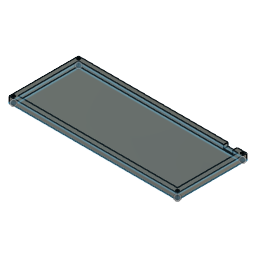
Keyboard Assembled (Autodesk Fusion 360 archive; units mm, degrees)
design "KeyboardBottom"
part number: 2026-01-12-19-14-13-415
Autodesk Fusion 360 part; units mm, degrees
(part 1 of 2)
sketch "Sketch1" plane through (0, 0, 0) normal (0, 0, 1) x (1, 0, 0)
  line L0 (0, 250) -> (351, 250)
  line L1 (351, 250) -> (351, 383)
  line L2 (351, 383) -> (0, 383)
  line L3 (0, 383) -> (0, 250)
  line L4 (-9.5, 392.5) -> (361.5, 392.5)
  line L5 (361.5, 392.5) -> (361.5, 239.5)
  line L6 (361.5, 239.5) -> (-9.5, 239.5)
  line L7 (-9.5, 239.5) -> (-9.5, 392.5)
  circle A0 centre (-4.5, 244.5) radius 1.7
  circle A1 centre (356.5, 244.5) radius 1.7
  circle A2 centre (-4.5, 387.5) radius 1.7
  circle A3 centre (356.5, 387.5) radius 1.7
  circle A4 centre (-4.5, 387.5) radius 3
  circle A5 centre (356.5, 244.5) radius 3
  circle A6 centre (-4.5, 244.5) radius 3
  circle A7 centre (356.5, 387.5) radius 3
  dimension "d1" = 351
  dimension "d2" = 133
  dimension "d3" = 371
  dimension "d4" = 153
  dimension "d5" = 9.5
  dimension "d10" = 9.5
  dimension "d11" = 3.4
  dimension "d12" = 5
  dimension "d13" = 5
  dimension "d14" = 3.4
  dimension "d15" = 5
  dimension "d16" = 5
  dimension "d17" = 3.4
  dimension "d18" = 5
  dimension "d19" = 5
  dimension "d21" = 5
  dimension "d22" = 5
  dimension "d23" = 6
  dimension "d24" = 6
  dimension "d25" = 6
  dimension "d26" = 6
  constraint horizontal L0
  constraint vertical L1
  constraint horizontal L2
  constraint vertical L3
  constraint horizontal L4
  constraint vertical L5
  constraint horizontal L6
  constraint vertical L7
  constraint coincident A2.centre A4.centre
  constraint coincident A0.centre A6.centre
  constraint coincident A1.centre A5.centre
  constraint coincident A3.centre A7.centre
  measures "d1" distance of L0.start L0.end
  measures "d2" distance of L0.start L2.end
  measures "d3" distance of L4.start L4.end
  measures "d4" distance of L4.start L6.end
  measures "d5" distance of L3 L7
  measures "d10" distance of L2 L4
  measures "d11" diameter of A0
  measures "d12" distance of L6 A0.centre
  measures "d13" distance of L7 A0.centre
  measures "d14" diameter of A1
  measures "d15" distance of L6 A1.centre
  measures "d16" distance of L5 A1.centre
  measures "d17" diameter of A2
  measures "d18" distance of L4 A2.centre
  measures "d19" distance of L7 A2.centre
  measures "d21" distance of L4 A3.centre
  measures "d22" distance of L5 A3.centre
  measures "d23" diameter of A4
  measures "d24" diameter of A5
  measures "d25" diameter of A6
  measures "d26" diameter of A7
extrude "Extrude1" add sketch "Sketch1" along normal blind 10 from surface at 3.1 contours A4 | A5 | A6 | A7 makes body 1 at (-1.5928, 245.2403, 9.7667) makes body 2 at (357.3125, 247.3879, 9.7667) makes body 3 at (-7.0599, 389.0643, 9.7667) makes body 4 at (355.1314, 384.8304, 6.4333)
extrude "Extrude2" add sketch "Sketch1" along normal blind 13 contours L4 L5 L6 L7 bodies 1 2 3 4
extrude "Extrude3" add sketch "Sketch1" along normal blind 3 contours L0 L1 L2 L3 bodies 1
sketch "Sketch2" plane through (0, 0, 13) normal (0, 0, 1) x (-1, 0, 0)
  line L0 (0, -250) -> (0, -383)
  line L1 (0, -383) -> (-351, -383)
  line L2 (-351, -383) -> (-351, -250)
  line L3 (-351, -250) -> (0, -250)
  circle A0 centre (-356.5, -244.5) radius 3
  circle A1 centre (4.5, -244.5) radius 3
  circle A2 centre (4.5, -387.5) radius 3
  circle A3 centre (-356.5, -387.5) radius 3
  line L4 (9.5, -239.5) -> (-361.5, -239.5)
  line L5 (-361.5, -239.5) -> (-361.5, -392.5)
  line L6 (-361.5, -392.5) -> (9.5, -392.5)
  line L7 (9.5, -392.5) -> (9.5, -239.5)
sketch "Sketch3" plane through (0, 0, 13) normal (0, 0, 1) x (-1, 0, 0)
  line L0 (2440, -1230) -> (2470, -1230)
  line L1 (2470, -1230) -> (2470, -1260)
  line L2 (2470, -1260) -> (2440, -1260)
  line L3 (2440, -1260) -> (2440, -1230)
  constraint horizontal L0
  constraint vertical L1
  constraint horizontal L2
  constraint vertical L3
sketch "Sketch4" plane through (0, 0, 0) normal (1, 0, 0) x (0, 1, 0)
sketch "Sketch5" plane through (0, 0, 0) normal (0, 0, 1) x (1, 0, 0)
extrude "Extrude4" cut sketch "Sketch3" against normal blind 7.5 bodies 1
sketch "Sketch6" plane through (0, 0, 13) normal (0, 0, 1) x (-1, 0, 0)
  line L0 (-320, -400) -> (-340, -400)
  line L1 (-340, -400) -> (-340, -380)
  line L2 (-340, -380) -> (-320, -380)
  line L3 (-320, -380) -> (-320, -400)
  constraint horizontal L0
  constraint vertical L1
  constraint horizontal L2
  constraint vertical L3
extrude "Extrude5" cut sketch "Sketch6" against normal blind 7.5 bodies 1

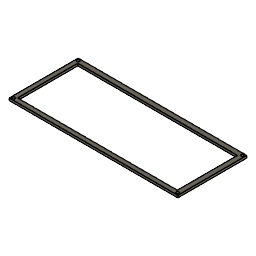
design "KeyboardBezel"
part number: 2026-01-27-16-23-20-670
Autodesk Fusion 360 part; units mm, degrees
sketch "Sketch1" plane through (0, 0, 0) normal (0, 0, 1) x (1, 0, 0)
  line L0 (0, 0) -> (-371, 0)
  line L1 (-371, 0) -> (-371, 152)
  line L2 (-371, 152) -> (0, 152)
  line L3 (0, 152) -> (0, 0)
  circle A0 centre (-366, 147) radius 1.7
  circle A1 centre (-5, 5) radius 1.7
  circle A2 centre (-366, 5) radius 1.7
  circle A3 centre (-5, 147) radius 1.7
  circle A4 centre (-366, 147) radius 3
  circle A5 centre (-5, 5) radius 3
  circle A6 centre (-366, 5) radius 3
  circle A7 centre (-5, 147) radius 3
  dimension "d1" = 371
  dimension "d2" = 152
  dimension "d3" = 3.4
  dimension "d4" = 5
  dimension "d5" = 5
  dimension "d6" = 3.4
  dimension "d7" = 3.4
  dimension "d8" = 3.4
  dimension "d9" = 5
  dimension "d10" = 5
  dimension "d11" = 5
  dimension "d12" = 5
  dimension "d13" = 5
  dimension "d14" = 5
  dimension "d15" = 6
  dimension "d16" = 6
  dimension "d17" = 6
  dimension "d18" = 6
  constraint horizontal L0
  constraint vertical L1
  constraint horizontal L2
  constraint vertical L3
  constraint coincident L0.start L3.end
  constraint coincident A1.centre A5.centre
  constraint coincident A3.centre A7.centre
  constraint coincident A0.centre A4.centre
  constraint coincident A2.centre A6.centre
  measures "d1" distance of L0.start L0.end
  measures "d2" distance of L0.start L2.end
  measures "d3" diameter of A0
  measures "d4" distance of L2 A0.centre
  measures "d5" distance of L1 A0.centre
  measures "d6" diameter of A1
  measures "d7" diameter of A2
  measures "d8" diameter of A3
  measures "d9" distance of L0 A2.centre
  measures "d10" distance of L1 A2.centre
  measures "d11" distance of L0 A1.centre
  measures "d12" distance of L3 A1.centre
  measures "d13" distance of L2 A3.centre
  measures "d14" distance of L3 A3.centre
  measures "d15" diameter of A4
  measures "d16" diameter of A5
  measures "d17" diameter of A6
  measures "d18" diameter of A7
sketch "Sketch2" plane through (0, 0, 0) normal (0, 0, 1) x (1, 0, 0)
  line L0 (-361.5, 141.5) -> (-10.5, 141.5)
  line L1 (-10.5, 141.5) -> (-10.5, 9.5)
  line L2 (-10.5, 9.5) -> (-361.5, 9.5)
  line L3 (-361.5, 9.5) -> (-361.5, 141.5)
  line L4 (0, 0) -> (-371, 0)
  line L5 (-371, 0) -> (-371, 152)
  dimension "d19" = 351
  dimension "d20" = 132
  dimension "d21" = 9.5
  dimension "d22" = 9.5
  constraint horizontal L0
  constraint vertical L1
  constraint horizontal L2
  constraint vertical L3
  measures "d19" distance of L0.start L0.end
  measures "d20" distance of L0.start L2.end
  measures "d21" distance of L2 L4
  measures "d22" distance of L3 L5
extrude "Extrude1" add sketch "Sketch1" along normal blind 5 contours L0 L1 L2 L3
extrude "Extrude2" cut sketch "Sketch2" along normal blind 10

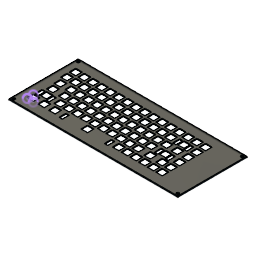
design "KeyboardPlate"
part number: 2026-01-21-16-41-26-618
Autodesk Fusion 360 part; units mm, degrees
sketch "plate-2026-01-22T00_34_46.063Z" plane through (0, 0, 0) normal (0, 0, 1) x (1, 0, 0)
  line L0 (3.025, -2.525) -> (16.025, -2.525)
  line L1 (3.025, -16.525) -> (16.025, -16.525)
  line L2 (2.525, -3.025) -> (2.525, -16.025)
  line L3 (16.525, -3.025) -> (16.525, -16.025)
  arc A0 (3.025, -2.525) -> (2.525, -3.025) centre (3.025, -3.025) ccw
  arc A1 (16.525, -3.025) -> (16.025, -2.525) centre (16.025, -3.025) ccw
  arc A2 (2.525, -16.025) -> (3.025, -16.525) centre (3.025, -16.025) ccw
  arc A3 (16.025, -16.525) -> (16.525, -16.025) centre (16.025, -16.025) ccw
  line L4 (22.075, -2.525) -> (35.075, -2.525)
  line L5 (22.075, -16.525) -> (35.075, -16.525)
  line L6 (21.575, -3.025) -> (21.575, -16.025)
  line L7 (35.575, -3.025) -> (35.575, -16.025)
  arc A4 (22.075, -2.525) -> (21.575, -3.025) centre (22.075, -3.025) ccw
  arc A5 (35.575, -3.025) -> (35.075, -2.525) centre (35.075, -3.025) ccw
  arc A6 (21.575, -16.025) -> (22.075, -16.525) centre (22.075, -16.025) ccw
  arc A7 (35.075, -16.525) -> (35.575, -16.025) centre (35.075, -16.025) ccw
  line L8 (41.125, -2.525) -> (54.125, -2.525)
  line L9 (41.125, -16.525) -> (54.125, -16.525)
  line L10 (40.625, -3.025) -> (40.625, -16.025)
  line L11 (54.625, -3.025) -> (54.625, -16.025)
  arc A8 (41.125, -2.525) -> (40.625, -3.025) centre (41.125, -3.025) ccw
  arc A9 (54.625, -3.025) -> (54.125, -2.525) centre (54.125, -3.025) ccw
  arc A10 (40.625, -16.025) -> (41.125, -16.525) centre (41.125, -16.025) ccw
  arc A11 (54.125, -16.525) -> (54.625, -16.025) centre (54.125, -16.025) ccw
  line L12 (60.175, -2.525) -> (73.175, -2.525)
  line L13 (60.175, -16.525) -> (73.175, -16.525)
  line L14 (59.675, -3.025) -> (59.675, -16.025)
  line L15 (73.675, -3.025) -> (73.675, -16.025)
  arc A12 (60.175, -2.525) -> (59.675, -3.025) centre (60.175, -3.025) ccw
  arc A13 (73.675, -3.025) -> (73.175, -2.525) centre (73.175, -3.025) ccw
  arc A14 (59.675, -16.025) -> (60.175, -16.525) centre (60.175, -16.025) ccw
  arc A15 (73.175, -16.525) -> (73.675, -16.025) centre (73.175, -16.025) ccw
  line L16 (79.225, -2.525) -> (92.225, -2.525)
  line L17 (79.225, -16.525) -> (92.225, -16.525)
  line L18 (78.725, -3.025) -> (78.725, -16.025)
  line L19 (92.725, -3.025) -> (92.725, -16.025)
  arc A16 (79.225, -2.525) -> (78.725, -3.025) centre (79.225, -3.025) ccw
  arc A17 (92.725, -3.025) -> (92.225, -2.525) centre (92.225, -3.025) ccw
  arc A18 (78.725, -16.025) -> (79.225, -16.525) centre (79.225, -16.025) ccw
  arc A19 (92.225, -16.525) -> (92.725, -16.025) centre (92.225, -16.025) ccw
  line L20 (98.275, -2.525) -> (111.275, -2.525)
  line L21 (98.275, -16.525) -> (111.275, -16.525)
  line L22 (97.775, -3.025) -> (97.775, -16.025)
  line L23 (111.775, -3.025) -> (111.775, -16.025)
  arc A20 (98.275, -2.525) -> (97.775, -3.025) centre (98.275, -3.025) ccw
  arc A21 (111.775, -3.025) -> (111.275, -2.525) centre (111.275, -3.025) ccw
  arc A22 (97.775, -16.025) -> (98.275, -16.525) centre (98.275, -16.025) ccw
  arc A23 (111.275, -16.525) -> (111.775, -16.025) centre (111.275, -16.025) ccw
  line L24 (117.325, -2.525) -> (130.325, -2.525)
  line L25 (117.325, -16.525) -> (130.325, -16.525)
  line L26 (116.825, -3.025) -> (116.825, -16.025)
  line L27 (130.825, -3.025) -> (130.825, -16.025)
  arc A24 (117.325, -2.525) -> (116.825, -3.025) centre (117.325, -3.025) ccw
  arc A25 (130.825, -3.025) -> (130.325, -2.525) centre (130.325, -3.025) ccw
  arc A26 (116.825, -16.025) -> (117.325, -16.525) centre (117.325, -16.025) ccw
  arc A27 (130.325, -16.525) -> (130.825, -16.025) centre (130.325, -16.025) ccw
  line L28 (136.375, -2.525) -> (149.375, -2.525)
  line L29 (136.375, -16.525) -> (149.375, -16.525)
  line L30 (135.875, -3.025) -> (135.875, -16.025)
  line L31 (149.875, -3.025) -> (149.875, -16.025)
  arc A28 (136.375, -2.525) -> (135.875, -3.025) centre (136.375, -3.025) ccw
  arc A29 (149.875, -3.025) -> (149.375, -2.525) centre (149.375, -3.025) ccw
  arc A30 (135.875, -16.025) -> (136.375, -16.525) centre (136.375, -16.025) ccw
  arc A31 (149.375, -16.525) -> (149.875, -16.025) centre (149.375, -16.025) ccw
  line L32 (155.425, -2.525) -> (168.425, -2.525)
  line L33 (155.425, -16.525) -> (168.425, -16.525)
  line L34 (154.925, -3.025) -> (154.925, -16.025)
  line L35 (168.925, -3.025) -> (168.925, -16.025)
  arc A32 (155.425, -2.525) -> (154.925, -3.025) centre (155.425, -3.025) ccw
  arc A33 (168.925, -3.025) -> (168.425, -2.525) centre (168.425, -3.025) ccw
  arc A34 (154.925, -16.025) -> (155.425, -16.525) centre (155.425, -16.025) ccw
  arc A35 (168.425, -16.525) -> (168.925, -16.025) centre (168.425, -16.025) ccw
  line L36 (174.475, -2.525) -> (187.475, -2.525)
  line L37 (174.475, -16.525) -> (187.475, -16.525)
  line L38 (173.975, -3.025) -> (173.975, -16.025)
  line L39 (187.975, -3.025) -> (187.975, -16.025)
  arc A36 (174.475, -2.525) -> (173.975, -3.025) centre (174.475, -3.025) ccw
  arc A37 (187.975, -3.025) -> (187.475, -2.525) centre (187.475, -3.025) ccw
  arc A38 (173.975, -16.025) -> (174.475, -16.525) centre (174.475, -16.025) ccw
  arc A39 (187.475, -16.525) -> (187.975, -16.025) centre (187.475, -16.025) ccw
  line L40 (193.525, -2.525) -> (206.525, -2.525)
  line L41 (193.525, -16.525) -> (206.525, -16.525)
  line L42 (193.025, -3.025) -> (193.025, -16.025)
  line L43 (207.025, -3.025) -> (207.025, -16.025)
  arc A40 (193.525, -2.525) -> (193.025, -3.025) centre (193.525, -3.025) ccw
  arc A41 (207.025, -3.025) -> (206.525, -2.525) centre (206.525, -3.025) ccw
  arc A42 (193.025, -16.025) -> (193.525, -16.525) centre (193.525, -16.025) ccw
  arc A43 (206.525, -16.525) -> (207.025, -16.025) centre (206.525, -16.025) ccw
  line L44 (212.575, -2.525) -> (225.575, -2.525)
  line L45 (212.575, -16.525) -> (225.575, -16.525)
  line L46 (212.075, -3.025) -> (212.075, -16.025)
  line L47 (226.075, -3.025) -> (226.075, -16.025)
  arc A44 (212.575, -2.525) -> (212.075, -3.025) centre (212.575, -3.025) ccw
  arc A45 (226.075, -3.025) -> (225.575, -2.525) centre (225.575, -3.025) ccw
  arc A46 (212.075, -16.025) -> (212.575, -16.525) centre (212.575, -16.025) ccw
  arc A47 (225.575, -16.525) -> (226.075, -16.025) centre (225.575, -16.025) ccw
  line L48 (231.625, -2.525) -> (244.625, -2.525)
  line L49 (231.625, -16.525) -> (244.625, -16.525)
  line L50 (231.125, -3.025) -> (231.125, -16.025)
  line L51 (245.125, -3.025) -> (245.125, -16.025)
  arc A48 (231.625, -2.525) -> (231.125, -3.025) centre (231.625, -3.025) ccw
  arc A49 (245.125, -3.025) -> (244.625, -2.525) centre (244.625, -3.025) ccw
  arc A50 (231.125, -16.025) -> (231.625, -16.525) centre (231.625, -16.025) ccw
  arc A51 (244.625, -16.525) -> (245.125, -16.025) centre (244.625, -16.025) ccw
  line L52 (250.675, -2.525) -> (263.675, -2.525)
  line L53 (250.675, -16.525) -> (263.675, -16.525)
  line L54 (250.175, -3.025) -> (250.175, -16.025)
  line L55 (264.175, -3.025) -> (264.175, -16.025)
  arc A52 (250.675, -2.525) -> (250.175, -3.025) centre (250.675, -3.025) ccw
  arc A53 (264.175, -3.025) -> (263.675, -2.525) centre (263.675, -3.025) ccw
  arc A54 (250.175, -16.025) -> (250.675, -16.525) centre (250.675, -16.025) ccw
  arc A55 (263.675, -16.525) -> (264.175, -16.025) centre (263.675, -16.025) ccw
  line L56 (269.725, -2.525) -> (282.725, -2.525)
  line L57 (269.725, -16.525) -> (282.725, -16.525)
  line L58 (269.225, -3.025) -> (269.225, -16.025)
  line L59 (283.225, -3.025) -> (283.225, -16.025)
  arc A56 (269.725, -2.525) -> (269.225, -3.025) centre (269.725, -3.025) ccw
  arc A57 (283.225, -3.025) -> (282.725, -2.525) centre (282.725, -3.025) ccw
  arc A58 (269.225, -16.025) -> (269.725, -16.525) centre (269.725, -16.025) ccw
  arc A59 (282.725, -16.525) -> (283.225, -16.025) centre (282.725, -16.025) ccw
  line L60 (288.775, -2.525) -> (301.775, -2.525)
  line L61 (288.775, -16.525) -> (301.775, -16.525)
  line L62 (288.275, -3.025) -> (288.275, -16.025)
  line L63 (302.275, -3.025) -> (302.275, -16.025)
  arc A60 (288.775, -2.525) -> (288.275, -3.025) centre (288.775, -3.025) ccw
  arc A61 (302.275, -3.025) -> (301.775, -2.525) centre (301.775, -3.025) ccw
  arc A62 (288.275, -16.025) -> (288.775, -16.525) centre (288.775, -16.025) ccw
  arc A63 (301.775, -16.525) -> (302.275, -16.025) centre (301.775, -16.025) ccw
  line L64 (3.025, -21.575) -> (16.025, -21.575)
  line L65 (3.025, -35.575) -> (16.025, -35.575)
  line L66 (2.525, -22.075) -> (2.525, -35.075)
  line L67 (16.525, -22.075) -> (16.525, -35.075)
  arc A64 (3.025, -21.575) -> (2.525, -22.075) centre (3.025, -22.075) ccw
  arc A65 (16.525, -22.075) -> (16.025, -21.575) centre (16.025, -22.075) ccw
  arc A66 (2.525, -35.075) -> (3.025, -35.575) centre (3.025, -35.075) ccw
  arc A67 (16.025, -35.575) -> (16.525, -35.075) centre (16.025, -35.075) ccw
  line L68 (22.075, -21.575) -> (35.075, -21.575)
  line L69 (22.075, -35.575) -> (35.075, -35.575)
  line L70 (21.575, -22.075) -> (21.575, -35.075)
  line L71 (35.575, -22.075) -> (35.575, -35.075)
  arc A68 (22.075, -21.575) -> (21.575, -22.075) centre (22.075, -22.075) ccw
  arc A69 (35.575, -22.075) -> (35.075, -21.575) centre (35.075, -22.075) ccw
  arc A70 (21.575, -35.075) -> (22.075, -35.575) centre (22.075, -35.075) ccw
  arc A71 (35.075, -35.575) -> (35.575, -35.075) centre (35.075, -35.075) ccw
  line L72 (41.125, -21.575) -> (54.125, -21.575)
  line L73 (41.125, -35.575) -> (54.125, -35.575)
  line L74 (40.625, -22.075) -> (40.625, -35.075)
  line L75 (54.625, -22.075) -> (54.625, -35.075)
  arc A72 (41.125, -21.575) -> (40.625, -22.075) centre (41.125, -22.075) ccw
  arc A73 (54.625, -22.075) -> (54.125, -21.575) centre (54.125, -22.075) ccw
  arc A74 (40.625, -35.075) -> (41.125, -35.575) centre (41.125, -35.075) ccw
  arc A75 (54.125, -35.575) -> (54.625, -35.075) centre (54.125, -35.075) ccw
  line L76 (60.175, -21.575) -> (73.175, -21.575)
  line L77 (60.175, -35.575) -> (73.175, -35.575)
  line L78 (59.675, -22.075) -> (59.675, -35.075)
  line L79 (73.675, -22.075) -> (73.675, -35.075)
  arc A76 (60.175, -21.575) -> (59.675, -22.075) centre (60.175, -22.075) ccw
  arc A77 (73.675, -22.075) -> (73.175, -21.575) centre (73.175, -22.075) ccw
  arc A78 (59.675, -35.075) -> (60.175, -35.575) centre (60.175, -35.075) ccw
  arc A79 (73.175, -35.575) -> (73.675, -35.075) centre (73.175, -35.075) ccw
  line L80 (79.225, -21.575) -> (92.225, -21.575)
  line L81 (79.225, -35.575) -> (92.225, -35.575)
  line L82 (78.725, -22.075) -> (78.725, -35.075)
  line L83 (92.725, -22.075) -> (92.725, -35.075)
  arc A80 (79.225, -21.575) -> (78.725, -22.075) centre (79.225, -22.075) ccw
  arc A81 (92.725, -22.075) -> (92.225, -21.575) centre (92.225, -22.075) ccw
  arc A82 (78.725, -35.075) -> (79.225, -35.575) centre (79.225, -35.075) ccw
  arc A83 (92.225, -35.575) -> (92.725, -35.075) centre (92.225, -35.075) ccw
  line L84 (98.275, -21.575) -> (111.275, -21.575)
  line L85 (98.275, -35.575) -> (111.275, -35.575)
  line L86 (97.775, -22.075) -> (97.775, -35.075)
  line L87 (111.775, -22.075) -> (111.775, -35.075)
  arc A84 (98.275, -21.575) -> (97.775, -22.075) centre (98.275, -22.075) ccw
  arc A85 (111.775, -22.075) -> (111.275, -21.575) centre (111.275, -22.075) ccw
  arc A86 (97.775, -35.075) -> (98.275, -35.575) centre (98.275, -35.075) ccw
  arc A87 (111.275, -35.575) -> (111.775, -35.075) centre (111.275, -35.075) ccw
  line L88 (117.325, -21.575) -> (130.325, -21.575)
  line L89 (117.325, -35.575) -> (130.325, -35.575)
  line L90 (116.825, -22.075) -> (116.825, -35.075)
  line L91 (130.825, -22.075) -> (130.825, -35.075)
  arc A88 (117.325, -21.575) -> (116.825, -22.075) centre (117.325, -22.075) ccw
  arc A89 (130.825, -22.075) -> (130.325, -21.575) centre (130.325, -22.075) ccw
  arc A90 (116.825, -35.075) -> (117.325, -35.575) centre (117.325, -35.075) ccw
  arc A91 (130.325, -35.575) -> (130.825, -35.075) centre (130.325, -35.075) ccw
  line L92 (136.375, -21.575) -> (149.375, -21.575)
  line L93 (136.375, -35.575) -> (149.375, -35.575)
  line L94 (135.875, -22.075) -> (135.875, -35.075)
  line L95 (149.875, -22.075) -> (149.875, -35.075)
  arc A92 (136.375, -21.575) -> (135.875, -22.075) centre (136.375, -22.075) ccw
  arc A93 (149.875, -22.075) -> (149.375, -21.575) centre (149.375, -22.075) ccw
  arc A94 (135.875, -35.075) -> (136.375, -35.575) centre (136.375, -35.075) ccw
  arc A95 (149.375, -35.575) -> (149.875, -35.075) centre (149.375, -35.075) ccw
  line L96 (155.425, -21.575) -> (168.425, -21.575)
  line L97 (155.425, -35.575) -> (168.425, -35.575)
  line L98 (154.925, -22.075) -> (154.925, -35.075)
  line L99 (168.925, -22.075) -> (168.925, -35.075)
  arc A96 (155.425, -21.575) -> (154.925, -22.075) centre (155.425, -22.075) ccw
  arc A97 (168.925, -22.075) -> (168.425, -21.575) centre (168.425, -22.075) ccw
  arc A98 (154.925, -35.075) -> (155.425, -35.575) centre (155.425, -35.075) ccw
  arc A99 (168.425, -35.575) -> (168.925, -35.075) centre (168.425, -35.075) ccw
  line L100 (174.475, -21.575) -> (187.475, -21.575)
  line L101 (174.475, -35.575) -> (187.475, -35.575)
  line L102 (173.975, -22.075) -> (173.975, -35.075)
  line L103 (187.975, -22.075) -> (187.975, -35.075)
  arc A100 (174.475, -21.575) -> (173.975, -22.075) centre (174.475, -22.075) ccw
  arc A101 (187.975, -22.075) -> (187.475, -21.575) centre (187.475, -22.075) ccw
  arc A102 (173.975, -35.075) -> (174.475, -35.575) centre (174.475, -35.075) ccw
  arc A103 (187.475, -35.575) -> (187.975, -35.075) centre (187.475, -35.075) ccw
  line L104 (193.525, -21.575) -> (206.525, -21.575)
  line L105 (193.525, -35.575) -> (206.525, -35.575)
  line L106 (193.025, -22.075) -> (193.025, -35.075)
  line L107 (207.025, -22.075) -> (207.025, -35.075)
  arc A104 (193.525, -21.575) -> (193.025, -22.075) centre (193.525, -22.075) ccw
  arc A105 (207.025, -22.075) -> (206.525, -21.575) centre (206.525, -22.075) ccw
  arc A106 (193.025, -35.075) -> (193.525, -35.575) centre (193.525, -35.075) ccw
  arc A107 (206.525, -35.575) -> (207.025, -35.075) centre (206.525, -35.075) ccw
  line L108 (212.575, -21.575) -> (225.575, -21.575)
  line L109 (212.575, -35.575) -> (225.575, -35.575)
  line L110 (212.075, -22.075) -> (212.075, -35.075)
  line L111 (226.075, -22.075) -> (226.075, -35.075)
  arc A108 (212.575, -21.575) -> (212.075, -22.075) centre (212.575, -22.075) ccw
  arc A109 (226.075, -22.075) -> (225.575, -21.575) centre (225.575, -22.075) ccw
  arc A110 (212.075, -35.075) -> (212.575, -35.575) centre (212.575, -35.075) ccw
  arc A111 (225.575, -35.575) -> (226.075, -35.075) centre (225.575, -35.075) ccw
  line L112 (231.625, -21.575) -> (244.625, -21.575)
  line L113 (231.625, -35.575) -> (244.625, -35.575)
  line L114 (231.125, -22.075) -> (231.125, -35.075)
  line L115 (245.125, -22.075) -> (245.125, -35.075)
  arc A112 (231.625, -21.575) -> (231.125, -22.075) centre (231.625, -22.075) ccw
  arc A113 (245.125, -22.075) -> (244.625, -21.575) centre (244.625, -22.075) ccw
  arc A114 (231.125, -35.075) -> (231.625, -35.575) centre (231.625, -35.075) ccw
  arc A115 (244.625, -35.575) -> (245.125, -35.075) centre (244.625, -35.075) ccw
  line L116 (260.2, -21.575) -> (273.2, -21.575)
  line L117 (260.2, -35.575) -> (273.2, -35.575)
  line L118 (259.7, -22.075) -> (259.7, -35.075)
  line L119 (273.7, -22.075) -> (273.7, -35.075)
  arc A116 (260.2, -21.575) -> (259.7, -22.075) centre (260.2, -22.075) ccw
  arc A117 (273.7, -22.075) -> (273.2, -21.575) centre (273.2, -22.075) ccw
  arc A118 (259.7, -35.075) -> (260.2, -35.575) centre (260.2, -35.075) ccw
  arc A119 (273.2, -35.575) -> (273.7, -35.075) centre (273.2, -35.075) ccw
  line L120 (251.762, -22.575) -> (257.762, -22.575)
  line L121 (251.762, -37.575) -> (257.762, -37.575)
  line L122 (251.262, -23.075) -> (251.262, -37.075)
  line L123 (258.262, -23.075) -> (258.262, -37.075)
  arc A120 (251.762, -22.575) -> (251.262, -23.075) centre (251.762, -23.075) ccw
  arc A121 (258.262, -23.075) -> (257.762, -22.575) centre (257.762, -23.075) ccw
  arc A122 (251.262, -37.075) -> (251.762, -37.575) centre (251.762, -37.075) ccw
  arc A123 (257.762, -37.575) -> (258.262, -37.075) centre (257.762, -37.075) ccw
  line L124 (275.638, -22.575) -> (281.638, -22.575)
  line L125 (275.638, -37.575) -> (281.638, -37.575)
  line L126 (275.138, -23.075) -> (275.138, -37.075)
  line L127 (282.138, -23.075) -> (282.138, -37.075)
  arc A124 (275.638, -22.575) -> (275.138, -23.075) centre (275.638, -23.075) ccw
  arc A125 (282.138, -23.075) -> (281.638, -22.575) centre (281.638, -23.075) ccw
  arc A126 (275.138, -37.075) -> (275.638, -37.575) centre (275.638, -37.075) ccw
  arc A127 (281.638, -37.575) -> (282.138, -37.075) centre (281.638, -37.075) ccw
  line L128 (288.775, -21.575) -> (301.775, -21.575)
  line L129 (288.775, -35.575) -> (301.775, -35.575)
  line L130 (288.275, -22.075) -> (288.275, -35.075)
  line L131 (302.275, -22.075) -> (302.275, -35.075)
  arc A128 (288.775, -21.575) -> (288.275, -22.075) centre (288.775, -22.075) ccw
  arc A129 (302.275, -22.075) -> (301.775, -21.575) centre (301.775, -22.075) ccw
  arc A130 (288.275, -35.075) -> (288.775, -35.575) centre (288.775, -35.075) ccw
  arc A131 (301.775, -35.575) -> (302.275, -35.075) centre (301.775, -35.075) ccw
  line L132 (7.7875, -40.625) -> (20.7875, -40.625)
  line L133 (7.7875, -54.625) -> (20.7875, -54.625)
  line L134 (7.2875, -41.125) -> (7.2875, -54.125)
  line L135 (21.2875, -41.125) -> (21.2875, -54.125)
  arc A132 (7.7875, -40.625) -> (7.2875, -41.125) centre (7.7875, -41.125) ccw
  arc A133 (21.2875, -41.125) -> (20.7875, -40.625) centre (20.7875, -41.125) ccw
  arc A134 (7.2875, -54.125) -> (7.7875, -54.625) centre (7.7875, -54.125) ccw
  arc A135 (20.7875, -54.625) -> (21.2875, -54.125) centre (20.7875, -54.125) ccw
  line L136 (31.6, -40.625) -> (44.6, -40.625)
  line L137 (31.6, -54.625) -> (44.6, -54.625)
  line L138 (31.1, -41.125) -> (31.1, -54.125)
  line L139 (45.1, -41.125) -> (45.1, -54.125)
  arc A136 (31.6, -40.625) -> (31.1, -41.125) centre (31.6, -41.125) ccw
  arc A137 (45.1, -41.125) -> (44.6, -40.625) centre (44.6, -41.125) ccw
  arc A138 (31.1, -54.125) -> (31.6, -54.625) centre (31.6, -54.125) ccw
  arc A139 (44.6, -54.625) -> (45.1, -54.125) centre (44.6, -54.125) ccw
  line L140 (50.65, -40.625) -> (63.65, -40.625)
  line L141 (50.65, -54.625) -> (63.65, -54.625)
  line L142 (50.15, -41.125) -> (50.15, -54.125)
  line L143 (64.15, -41.125) -> (64.15, -54.125)
  arc A140 (50.65, -40.625) -> (50.15, -41.125) centre (50.65, -41.125) ccw
  arc A141 (64.15, -41.125) -> (63.65, -40.625) centre (63.65, -41.125) ccw
  arc A142 (50.15, -54.125) -> (50.65, -54.625) centre (50.65, -54.125) ccw
  arc A143 (63.65, -54.625) -> (64.15, -54.125) centre (63.65, -54.125) ccw
  line L144 (69.7, -40.625) -> (82.7, -40.625)
  line L145 (69.7, -54.625) -> (82.7, -54.625)
  line L146 (69.2, -41.125) -> (69.2, -54.125)
  line L147 (83.2, -41.125) -> (83.2, -54.125)
  arc A144 (69.7, -40.625) -> (69.2, -41.125) centre (69.7, -41.125) ccw
  arc A145 (83.2, -41.125) -> (82.7, -40.625) centre (82.7, -41.125) ccw
  arc A146 (69.2, -54.125) -> (69.7, -54.625) centre (69.7, -54.125) ccw
  arc A147 (82.7, -54.625) -> (83.2, -54.125) centre (82.7, -54.125) ccw
  line L148 (88.75, -40.625) -> (101.75, -40.625)
  line L149 (88.75, -54.625) -> (101.75, -54.625)
  line L150 (88.25, -41.125) -> (88.25, -54.125)
  line L151 (102.25, -41.125) -> (102.25, -54.125)
  arc A148 (88.75, -40.625) -> (88.25, -41.125) centre (88.75, -41.125) ccw
  arc A149 (102.25, -41.125) -> (101.75, -40.625) centre (101.75, -41.125) ccw
  arc A150 (88.25, -54.125) -> (88.75, -54.625) centre (88.75, -54.125) ccw
  arc A151 (101.75, -54.625) -> (102.25, -54.125) centre (101.75, -54.125) ccw
  line L152 (107.8, -40.625) -> (120.8, -40.625)
  line L153 (107.8, -54.625) -> (120.8, -54.625)
  line L154 (107.3, -41.125) -> (107.3, -54.125)
  line L155 (121.3, -41.125) -> (121.3, -54.125)
  arc A152 (107.8, -40.625) -> (107.3, -41.125) centre (107.8, -41.125) ccw
  arc A153 (121.3, -41.125) -> (120.8, -40.625) centre (120.8, -41.125) ccw
  arc A154 (107.3, -54.125) -> (107.8, -54.625) centre (107.8, -54.125) ccw
  arc A155 (120.8, -54.625) -> (121.3, -54.125) centre (120.8, -54.125) ccw
  line L156 (126.85, -40.625) -> (139.85, -40.625)
  line L157 (126.85, -54.625) -> (139.85, -54.625)
  line L158 (126.35, -41.125) -> (126.35, -54.125)
  line L159 (140.35, -41.125) -> (140.35, -54.125)
  arc A156 (126.85, -40.625) -> (126.35, -41.125) centre (126.85, -41.125) ccw
  arc A157 (140.35, -41.125) -> (139.85, -40.625) centre (139.85, -41.125) ccw
  arc A158 (126.35, -54.125) -> (126.85, -54.625) centre (126.85, -54.125) ccw
  arc A159 (139.85, -54.625) -> (140.35, -54.125) centre (139.85, -54.125) ccw
  line L160 (145.9, -40.625) -> (158.9, -40.625)
  line L161 (145.9, -54.625) -> (158.9, -54.625)
  line L162 (145.4, -41.125) -> (145.4, -54.125)
  line L163 (159.4, -41.125) -> (159.4, -54.125)
  arc A160 (145.9, -40.625) -> (145.4, -41.125) centre (145.9, -41.125) ccw
  arc A161 (159.4, -41.125) -> (158.9, -40.625) centre (158.9, -41.125) ccw
  arc A162 (145.4, -54.125) -> (145.9, -54.625) centre (145.9, -54.125) ccw
  arc A163 (158.9, -54.625) -> (159.4, -54.125) centre (158.9, -54.125) ccw
  line L164 (164.95, -40.625) -> (177.95, -40.625)
  line L165 (164.95, -54.625) -> (177.95, -54.625)
  line L166 (164.45, -41.125) -> (164.45, -54.125)
  line L167 (178.45, -41.125) -> (178.45, -54.125)
  arc A164 (164.95, -40.625) -> (164.45, -41.125) centre (164.95, -41.125) ccw
  arc A165 (178.45, -41.125) -> (177.95, -40.625) centre (177.95, -41.125) ccw
  arc A166 (164.45, -54.125) -> (164.95, -54.625) centre (164.95, -54.125) ccw
  arc A167 (177.95, -54.625) -> (178.45, -54.125) centre (177.95, -54.125) ccw
  line L168 (184, -40.625) -> (197, -40.625)
  line L169 (184, -54.625) -> (197, -54.625)
  line L170 (183.5, -41.125) -> (183.5, -54.125)
  line L171 (197.5, -41.125) -> (197.5, -54.125)
  arc A168 (184, -40.625) -> (183.5, -41.125) centre (184, -41.125) ccw
  arc A169 (197.5, -41.125) -> (197, -40.625) centre (197, -41.125) ccw
  arc A170 (183.5, -54.125) -> (184, -54.625) centre (184, -54.125) ccw
  arc A171 (197, -54.625) -> (197.5, -54.125) centre (197, -54.125) ccw
  line L172 (203.05, -40.625) -> (216.05, -40.625)
  line L173 (203.05, -54.625) -> (216.05, -54.625)
  line L174 (202.55, -41.125) -> (202.55, -54.125)
  line L175 (216.55, -41.125) -> (216.55, -54.125)
  arc A172 (203.05, -40.625) -> (202.55, -41.125) centre (203.05, -41.125) ccw
  arc A173 (216.55, -41.125) -> (216.05, -40.625) centre (216.05, -41.125) ccw
  arc A174 (202.55, -54.125) -> (203.05, -54.625) centre (203.05, -54.125) ccw
  arc A175 (216.05, -54.625) -> (216.55, -54.125) centre (216.05, -54.125) ccw
  line L176 (222.1, -40.625) -> (235.1, -40.625)
  line L177 (222.1, -54.625) -> (235.1, -54.625)
  line L178 (221.6, -41.125) -> (221.6, -54.125)
  line L179 (235.6, -41.125) -> (235.6, -54.125)
  arc A176 (222.1, -40.625) -> (221.6, -41.125) centre (222.1, -41.125) ccw
  arc A177 (235.6, -41.125) -> (235.1, -40.625) centre (235.1, -41.125) ccw
  arc A178 (221.6, -54.125) -> (222.1, -54.625) centre (222.1, -54.125) ccw
  arc A179 (235.1, -54.625) -> (235.6, -54.125) centre (235.1, -54.125) ccw
  line L180 (241.15, -40.625) -> (254.15, -40.625)
  line L181 (241.15, -54.625) -> (254.15, -54.625)
  line L182 (240.65, -41.125) -> (240.65, -54.125)
  line L183 (254.65, -41.125) -> (254.65, -54.125)
  arc A180 (241.15, -40.625) -> (240.65, -41.125) centre (241.15, -41.125) ccw
  arc A181 (254.65, -41.125) -> (254.15, -40.625) centre (254.15, -41.125) ccw
  arc A182 (240.65, -54.125) -> (241.15, -54.625) centre (241.15, -54.125) ccw
  arc A183 (254.15, -54.625) -> (254.65, -54.125) centre (254.15, -54.125) ccw
  line L184 (264.9625, -40.625) -> (277.9625, -40.625)
  line L185 (264.9625, -54.625) -> (277.9625, -54.625)
  line L186 (264.4625, -41.125) -> (264.4625, -54.125)
  line L187 (278.4625, -41.125) -> (278.4625, -54.125)
  arc A184 (264.9625, -40.625) -> (264.4625, -41.125) centre (264.9625, -41.125) ccw
  arc A185 (278.4625, -41.125) -> (277.9625, -40.625) centre (277.9625, -41.125) ccw
  arc A186 (264.4625, -54.125) -> (264.9625, -54.625) centre (264.9625, -54.125) ccw
  arc A187 (277.9625, -54.625) -> (278.4625, -54.125) centre (277.9625, -54.125) ccw
  line L188 (288.775, -40.625) -> (301.775, -40.625)
  line L189 (288.775, -54.625) -> (301.775, -54.625)
  line L190 (288.275, -41.125) -> (288.275, -54.125)
  line L191 (302.275, -41.125) -> (302.275, -54.125)
  arc A188 (288.775, -40.625) -> (288.275, -41.125) centre (288.775, -41.125) ccw
  arc A189 (302.275, -41.125) -> (301.775, -40.625) centre (301.775, -41.125) ccw
  arc A190 (288.275, -54.125) -> (288.775, -54.625) centre (288.775, -54.125) ccw
  arc A191 (301.775, -54.625) -> (302.275, -54.125) centre (301.775, -54.125) ccw
  line L192 (10.1687, -59.675) -> (23.1687, -59.675)
  line L193 (10.1687, -73.675) -> (23.1687, -73.675)
  line L194 (9.6687, -60.175) -> (9.6687, -73.175)
  line L195 (23.6687, -60.175) -> (23.6687, -73.175)
  arc A192 (10.1687, -59.675) -> (9.6688, -60.175) centre (10.1687, -60.175) ccw
  arc A193 (23.6687, -60.175) -> (23.1687, -59.675) centre (23.1687, -60.175) ccw
  arc A194 (9.6687, -73.175) -> (10.1687, -73.675) centre (10.1687, -73.175) ccw
  arc A195 (23.1687, -73.675) -> (23.6687, -73.175) centre (23.1687, -73.175) ccw
  line L196 (36.3625, -59.675) -> (49.3625, -59.675)
  line L197 (36.3625, -73.675) -> (49.3625, -73.675)
  line L198 (35.8625, -60.175) -> (35.8625, -73.175)
  line L199 (49.8625, -60.175) -> (49.8625, -73.175)
  arc A196 (36.3625, -59.675) -> (35.8625, -60.175) centre (36.3625, -60.175) ccw
  arc A197 (49.8625, -60.175) -> (49.3625, -59.675) centre (49.3625, -60.175) ccw
  arc A198 (35.8625, -73.175) -> (36.3625, -73.675) centre (36.3625, -73.175) ccw
  arc A199 (49.3625, -73.675) -> (49.8625, -73.175) centre (49.3625, -73.175) ccw
  line L200 (55.4125, -59.675) -> (68.4125, -59.675)
  line L201 (55.4125, -73.675) -> (68.4125, -73.675)
  line L202 (54.9125, -60.175) -> (54.9125, -73.175)
  line L203 (68.9125, -60.175) -> (68.9125, -73.175)
  arc A200 (55.4125, -59.675) -> (54.9125, -60.175) centre (55.4125, -60.175) ccw
  arc A201 (68.9125, -60.175) -> (68.4125, -59.675) centre (68.4125, -60.175) ccw
  arc A202 (54.9125, -73.175) -> (55.4125, -73.675) centre (55.4125, -73.175) ccw
  arc A203 (68.4125, -73.675) -> (68.9125, -73.175) centre (68.4125, -73.175) ccw
  line L204 (74.4625, -59.675) -> (87.4625, -59.675)
  line L205 (74.4625, -73.675) -> (87.4625, -73.675)
  line L206 (73.9625, -60.175) -> (73.9625, -73.175)
  line L207 (87.9625, -60.175) -> (87.9625, -73.175)
  arc A204 (74.4625, -59.675) -> (73.9625, -60.175) centre (74.4625, -60.175) ccw
  arc A205 (87.9625, -60.175) -> (87.4625, -59.675) centre (87.4625, -60.175) ccw
  arc A206 (73.9625, -73.175) -> (74.4625, -73.675) centre (74.4625, -73.175) ccw
  arc A207 (87.4625, -73.675) -> (87.9625, -73.175) centre (87.4625, -73.175) ccw
  line L208 (93.5125, -59.675) -> (106.5125, -59.675)
  line L209 (93.5125, -73.675) -> (106.5125, -73.675)
  line L210 (93.0125, -60.175) -> (93.0125, -73.175)
  line L211 (107.0125, -60.175) -> (107.0125, -73.175)
  arc A208 (93.5125, -59.675) -> (93.0125, -60.175) centre (93.5125, -60.175) ccw
  arc A209 (107.0125, -60.175) -> (106.5125, -59.675) centre (106.5125, -60.175) ccw
  arc A210 (93.0125, -73.175) -> (93.5125, -73.675) centre (93.5125, -73.175) ccw
  arc A211 (106.5125, -73.675) -> (107.0125, -73.175) centre (106.5125, -73.175) ccw
  line L212 (112.5625, -59.675) -> (125.5625, -59.675)
  line L213 (112.5625, -73.675) -> (125.5625, -73.675)
  line L214 (112.0625, -60.175) -> (112.0625, -73.175)
  line L215 (126.0625, -60.175) -> (126.0625, -73.175)
  arc A212 (112.5625, -59.675) -> (112.0625, -60.175) centre (112.5625, -60.175) ccw
  arc A213 (126.0625, -60.175) -> (125.5625, -59.675) centre (125.5625, -60.175) ccw
  arc A214 (112.0625, -73.175) -> (112.5625, -73.675) centre (112.5625, -73.175) ccw
  arc A215 (125.5625, -73.675) -> (126.0625, -73.175) centre (125.5625, -73.175) ccw
  line L216 (131.6125, -59.675) -> (144.6125, -59.675)
  line L217 (131.6125, -73.675) -> (144.6125, -73.675)
  line L218 (131.1125, -60.175) -> (131.1125, -73.175)
  line L219 (145.1125, -60.175) -> (145.1125, -73.175)
  arc A216 (131.6125, -59.675) -> (131.1125, -60.175) centre (131.6125, -60.175) ccw
  arc A217 (145.1125, -60.175) -> (144.6125, -59.675) centre (144.6125, -60.175) ccw
  arc A218 (131.1125, -73.175) -> (131.6125, -73.675) centre (131.6125, -73.175) ccw
  arc A219 (144.6125, -73.675) -> (145.1125, -73.175) centre (144.6125, -73.175) ccw
  line L220 (150.6625, -59.675) -> (163.6625, -59.675)
  line L221 (150.6625, -73.675) -> (163.6625, -73.675)
  line L222 (150.1625, -60.175) -> (150.1625, -73.175)
  line L223 (164.1625, -60.175) -> (164.1625, -73.175)
  arc A220 (150.6625, -59.675) -> (150.1625, -60.175) centre (150.6625, -60.175) ccw
  arc A221 (164.1625, -60.175) -> (163.6625, -59.675) centre (163.6625, -60.175) ccw
  arc A222 (150.1625, -73.175) -> (150.6625, -73.675) centre (150.6625, -73.175) ccw
  arc A223 (163.6625, -73.675) -> (164.1625, -73.175) centre (163.6625, -73.175) ccw
  line L224 (169.7125, -59.675) -> (182.7125, -59.675)
  line L225 (169.7125, -73.675) -> (182.7125, -73.675)
  line L226 (169.2125, -60.175) -> (169.2125, -73.175)
  line L227 (183.2125, -60.175) -> (183.2125, -73.175)
  arc A224 (169.7125, -59.675) -> (169.2125, -60.175) centre (169.7125, -60.175) ccw
  arc A225 (183.2125, -60.175) -> (182.7125, -59.675) centre (182.7125, -60.175) ccw
  arc A226 (169.2125, -73.175) -> (169.7125, -73.675) centre (169.7125, -73.175) ccw
  arc A227 (182.7125, -73.675) -> (183.2125, -73.175) centre (182.7125, -73.175) ccw
  line L228 (188.7625, -59.675) -> (201.7625, -59.675)
  line L229 (188.7625, -73.675) -> (201.7625, -73.675)
  line L230 (188.2625, -60.175) -> (188.2625, -73.175)
  line L231 (202.2625, -60.175) -> (202.2625, -73.175)
  arc A228 (188.7625, -59.675) -> (188.2625, -60.175) centre (188.7625, -60.175) ccw
  arc A229 (202.2625, -60.175) -> (201.7625, -59.675) centre (201.7625, -60.175) ccw
  arc A230 (188.2625, -73.175) -> (188.7625, -73.675) centre (188.7625, -73.175) ccw
  arc A231 (201.7625, -73.675) -> (202.2625, -73.175) centre (201.7625, -73.175) ccw
  line L232 (207.8125, -59.675) -> (220.8125, -59.675)
  line L233 (207.8125, -73.675) -> (220.8125, -73.675)
  line L234 (207.3125, -60.175) -> (207.3125, -73.175)
  line L235 (221.3125, -60.175) -> (221.3125, -73.175)
  arc A232 (207.8125, -59.675) -> (207.3125, -60.175) centre (207.8125, -60.175) ccw
  arc A233 (221.3125, -60.175) -> (220.8125, -59.675) centre (220.8125, -60.175) ccw
  arc A234 (207.3125, -73.175) -> (207.8125, -73.675) centre (207.8125, -73.175) ccw
  arc A235 (220.8125, -73.675) -> (221.3125, -73.175) centre (220.8125, -73.175) ccw
  line L236 (226.8625, -59.675) -> (239.8625, -59.675)
  line L237 (226.8625, -73.675) -> (239.8625, -73.675)
  line L238 (226.3625, -60.175) -> (226.3625, -73.175)
  line L239 (240.3625, -60.175) -> (240.3625, -73.175)
  arc A236 (226.8625, -59.675) -> (226.3625, -60.175) centre (226.8625, -60.175) ccw
  arc A237 (240.3625, -60.175) -> (239.8625, -59.675) centre (239.8625, -60.175) ccw
  arc A238 (226.3625, -73.175) -> (226.8625, -73.675) centre (226.8625, -73.175) ccw
  arc A239 (239.8625, -73.675) -> (240.3625, -73.175) centre (239.8625, -73.175) ccw
  line L240 (257.8188, -59.675) -> (270.8188, -59.675)
  line L241 (257.8188, -73.675) -> (270.8188, -73.675)
  line L242 (257.3188, -60.175) -> (257.3188, -73.175)
  line L243 (271.3188, -60.175) -> (271.3188, -73.175)
  arc A240 (257.8188, -59.675) -> (257.3188, -60.175) centre (257.8188, -60.175) ccw
  arc A241 (271.3188, -60.175) -> (270.8188, -59.675) centre (270.8188, -60.175) ccw
  arc A242 (257.3188, -73.175) -> (257.8188, -73.675) centre (257.8188, -73.175) ccw
  arc A243 (270.8188, -73.675) -> (271.3188, -73.175) centre (270.8188, -73.175) ccw
  line L244 (249.3808, -60.675) -> (255.3808, -60.675)
  line L245 (249.3808, -75.675) -> (255.3808, -75.675)
  line L246 (248.8808, -61.175) -> (248.8808, -75.175)
  line L247 (255.8808, -61.175) -> (255.8808, -75.175)
  arc A244 (249.3808, -60.675) -> (248.8808, -61.175) centre (249.3808, -61.175) ccw
  arc A245 (255.8808, -61.175) -> (255.3808, -60.675) centre (255.3808, -61.175) ccw
  arc A246 (248.8808, -75.175) -> (249.3808, -75.675) centre (249.3808, -75.175) ccw
  arc A247 (255.3808, -75.675) -> (255.8808, -75.175) centre (255.3808, -75.175) ccw
  line L248 (273.2568, -60.675) -> (279.2568, -60.675)
  line L249 (273.2568, -75.675) -> (279.2568, -75.675)
  line L250 (272.7568, -61.175) -> (272.7568, -75.175)
  line L251 (279.7568, -61.175) -> (279.7568, -75.175)
  arc A248 (273.2568, -60.675) -> (272.7568, -61.175) centre (273.2568, -61.175) ccw
  arc A249 (279.7568, -61.175) -> (279.2568, -60.675) centre (279.2568, -61.175) ccw
  arc A250 (272.7568, -75.175) -> (273.2568, -75.675) centre (273.2568, -75.175) ccw
  arc A251 (279.2568, -75.675) -> (279.7568, -75.175) centre (279.2568, -75.175) ccw
  line L252 (288.775, -59.675) -> (301.775, -59.675)
  line L253 (288.775, -73.675) -> (301.775, -73.675)
  line L254 (288.275, -60.175) -> (288.275, -73.175)
  line L255 (302.275, -60.175) -> (302.275, -73.175)
  arc A252 (288.775, -59.675) -> (288.275, -60.175) centre (288.775, -60.175) ccw
  arc A253 (302.275, -60.175) -> (301.775, -59.675) centre (301.775, -60.175) ccw
  arc A254 (288.275, -73.175) -> (288.775, -73.675) centre (288.775, -73.175) ccw
  arc A255 (301.775, -73.675) -> (302.275, -73.175) centre (301.775, -73.175) ccw
  line L256 (14.9313, -78.725) -> (27.9312, -78.725)
  line L257 (14.9313, -92.725) -> (27.9312, -92.725)
  line L258 (14.4313, -79.225) -> (14.4313, -92.225)
  line L259 (28.4313, -79.225) -> (28.4313, -92.225)
  arc A256 (14.9313, -78.725) -> (14.4313, -79.225) centre (14.9313, -79.225) ccw
  arc A257 (28.4313, -79.225) -> (27.9312, -78.725) centre (27.9312, -79.225) ccw
  arc A258 (14.4313, -92.225) -> (14.9313, -92.725) centre (14.9313, -92.225) ccw
  arc A259 (27.9312, -92.725) -> (28.4312, -92.225) centre (27.9312, -92.225) ccw
  line L260 (6.4933, -79.725) -> (12.4932, -79.725)
  line L261 (6.4933, -94.725) -> (12.4932, -94.725)
  line L262 (5.9932, -80.225) -> (5.9932, -94.225)
  line L263 (12.9932, -80.225) -> (12.9932, -94.225)
  arc A260 (6.4933, -79.725) -> (5.9933, -80.225) centre (6.4933, -80.225) ccw
  arc A261 (12.9932, -80.225) -> (12.4932, -79.725) centre (12.4932, -80.225) ccw
  arc A262 (5.9932, -94.225) -> (6.4933, -94.725) centre (6.4933, -94.225) ccw
  arc A263 (12.4932, -94.725) -> (12.9933, -94.225) centre (12.4932, -94.225) ccw
  line L264 (30.3693, -79.725) -> (36.3693, -79.725)
  line L265 (30.3693, -94.725) -> (36.3693, -94.725)
  line L266 (29.8693, -80.225) -> (29.8693, -94.225)
  line L267 (36.8693, -80.225) -> (36.8693, -94.225)
  arc A264 (30.3693, -79.725) -> (29.8693, -80.225) centre (30.3693, -80.225) ccw
  arc A265 (36.8693, -80.225) -> (36.3693, -79.725) centre (36.3693, -80.225) ccw
  arc A266 (29.8693, -94.225) -> (30.3693, -94.725) centre (30.3693, -94.225) ccw
  arc A267 (36.3693, -94.725) -> (36.8693, -94.225) centre (36.3693, -94.225) ccw
  line L268 (45.8875, -78.725) -> (58.8875, -78.725)
  line L269 (45.8875, -92.725) -> (58.8875, -92.725)
  line L270 (45.3875, -79.225) -> (45.3875, -92.225)
  line L271 (59.3875, -79.225) -> (59.3875, -92.225)
  arc A268 (45.8875, -78.725) -> (45.3875, -79.225) centre (45.8875, -79.225) ccw
  arc A269 (59.3875, -79.225) -> (58.8875, -78.725) centre (58.8875, -79.225) ccw
  arc A270 (45.3875, -92.225) -> (45.8875, -92.725) centre (45.8875, -92.225) ccw
  arc A271 (58.8875, -92.725) -> (59.3875, -92.225) centre (58.8875, -92.225) ccw
  line L272 (64.9375, -78.725) -> (77.9375, -78.725)
  line L273 (64.9375, -92.725) -> (77.9375, -92.725)
  line L274 (64.4375, -79.225) -> (64.4375, -92.225)
  line L275 (78.4375, -79.225) -> (78.4375, -92.225)
  arc A272 (64.9375, -78.725) -> (64.4375, -79.225) centre (64.9375, -79.225) ccw
  arc A273 (78.4375, -79.225) -> (77.9375, -78.725) centre (77.9375, -79.225) ccw
  arc A274 (64.4375, -92.225) -> (64.9375, -92.725) centre (64.9375, -92.225) ccw
  arc A275 (77.9375, -92.725) -> (78.4375, -92.225) centre (77.9375, -92.225) ccw
  line L276 (83.9875, -78.725) -> (96.9875, -78.725)
  line L277 (83.9875, -92.725) -> (96.9875, -92.725)
  line L278 (83.4875, -79.225) -> (83.4875, -92.225)
  line L279 (97.4875, -79.225) -> (97.4875, -92.225)
  arc A276 (83.9875, -78.725) -> (83.4875, -79.225) centre (83.9875, -79.225) ccw
  arc A277 (97.4875, -79.225) -> (96.9875, -78.725) centre (96.9875, -79.225) ccw
  arc A278 (83.4875, -92.225) -> (83.9875, -92.725) centre (83.9875, -92.225) ccw
  arc A279 (96.9875, -92.725) -> (97.4875, -92.225) centre (96.9875, -92.225) ccw
  line L280 (103.0375, -78.725) -> (116.0375, -78.725)
  line L281 (103.0375, -92.725) -> (116.0375, -92.725)
  line L282 (102.5375, -79.225) -> (102.5375, -92.225)
  line L283 (116.5375, -79.225) -> (116.5375, -92.225)
  arc A280 (103.0375, -78.725) -> (102.5375, -79.225) centre (103.0375, -79.225) ccw
  arc A281 (116.5375, -79.225) -> (116.0375, -78.725) centre (116.0375, -79.225) ccw
  arc A282 (102.5375, -92.225) -> (103.0375, -92.725) centre (103.0375, -92.225) ccw
  arc A283 (116.0375, -92.725) -> (116.5375, -92.225) centre (116.0375, -92.225) ccw
  line L284 (122.0875, -78.725) -> (135.0875, -78.725)
  line L285 (122.0875, -92.725) -> (135.0875, -92.725)
  line L286 (121.5875, -79.225) -> (121.5875, -92.225)
  line L287 (135.5875, -79.225) -> (135.5875, -92.225)
  arc A284 (122.0875, -78.725) -> (121.5875, -79.225) centre (122.0875, -79.225) ccw
  arc A285 (135.5875, -79.225) -> (135.0875, -78.725) centre (135.0875, -79.225) ccw
  arc A286 (121.5875, -92.225) -> (122.0875, -92.725) centre (122.0875, -92.225) ccw
  arc A287 (135.0875, -92.725) -> (135.5875, -92.225) centre (135.0875, -92.225) ccw
  line L288 (141.1375, -78.725) -> (154.1375, -78.725)
  line L289 (141.1375, -92.725) -> (154.1375, -92.725)
  line L290 (140.6375, -79.225) -> (140.6375, -92.225)
  line L291 (154.6375, -79.225) -> (154.6375, -92.225)
  arc A288 (141.1375, -78.725) -> (140.6375, -79.225) centre (141.1375, -79.225) ccw
  arc A289 (154.6375, -79.225) -> (154.1375, -78.725) centre (154.1375, -79.225) ccw
  arc A290 (140.6375, -92.225) -> (141.1375, -92.725) centre (141.1375, -92.225) ccw
  arc A291 (154.1375, -92.725) -> (154.6375, -92.225) centre (154.1375, -92.225) ccw
  line L292 (160.1875, -78.725) -> (173.1875, -78.725)
  line L293 (160.1875, -92.725) -> (173.1875, -92.725)
  line L294 (159.6875, -79.225) -> (159.6875, -92.225)
  line L295 (173.6875, -79.225) -> (173.6875, -92.225)
  arc A292 (160.1875, -78.725) -> (159.6875, -79.225) centre (160.1875, -79.225) ccw
  arc A293 (173.6875, -79.225) -> (173.1875, -78.725) centre (173.1875, -79.225) ccw
  arc A294 (159.6875, -92.225) -> (160.1875, -92.725) centre (160.1875, -92.225) ccw
  arc A295 (173.1875, -92.725) -> (173.6875, -92.225) centre (173.1875, -92.225) ccw
  line L296 (179.2375, -78.725) -> (192.2375, -78.725)
  line L297 (179.2375, -92.725) -> (192.2375, -92.725)
  line L298 (178.7375, -79.225) -> (178.7375, -92.225)
  line L299 (192.7375, -79.225) -> (192.7375, -92.225)
  arc A296 (179.2375, -78.725) -> (178.7375, -79.225) centre (179.2375, -79.225) ccw
  arc A297 (192.7375, -79.225) -> (192.2375, -78.725) centre (192.2375, -79.225) ccw
  arc A298 (178.7375, -92.225) -> (179.2375, -92.725) centre (179.2375, -92.225) ccw
  arc A299 (192.2375, -92.725) -> (192.7375, -92.225) centre (192.2375, -92.225) ccw
  line L300 (198.2875, -78.725) -> (211.2875, -78.725)
  line L301 (198.2875, -92.725) -> (211.2875, -92.725)
  line L302 (197.7875, -79.225) -> (197.7875, -92.225)
  line L303 (211.7875, -79.225) -> (211.7875, -92.225)
  arc A300 (198.2875, -78.725) -> (197.7875, -79.225) centre (198.2875, -79.225) ccw
  arc A301 (211.7875, -79.225) -> (211.2875, -78.725) centre (211.2875, -79.225) ccw
  arc A302 (197.7875, -92.225) -> (198.2875, -92.725) centre (198.2875, -92.225) ccw
  arc A303 (211.2875, -92.725) -> (211.7875, -92.225) centre (211.2875, -92.225) ccw
  line L304 (217.3375, -78.725) -> (230.3375, -78.725)
  line L305 (217.3375, -92.725) -> (230.3375, -92.725)
  line L306 (216.8375, -79.225) -> (216.8375, -92.225)
  line L307 (230.8375, -79.225) -> (230.8375, -92.225)
  arc A304 (217.3375, -78.725) -> (216.8375, -79.225) centre (217.3375, -79.225) ccw
  arc A305 (230.8375, -79.225) -> (230.3375, -78.725) centre (230.3375, -79.225) ccw
  arc A306 (216.8375, -92.225) -> (217.3375, -92.725) centre (217.3375, -92.225) ccw
  arc A307 (230.3375, -92.725) -> (230.8375, -92.225) centre (230.3375, -92.225) ccw
  line L308 (243.5313, -78.725) -> (256.5313, -78.725)
  line L309 (243.5313, -92.725) -> (256.5313, -92.725)
  line L310 (243.0312, -79.225) -> (243.0312, -92.225)
  line L311 (257.0312, -79.225) -> (257.0312, -92.225)
  arc A308 (243.5313, -78.725) -> (243.0313, -79.225) centre (243.5313, -79.225) ccw
  arc A309 (257.0312, -79.225) -> (256.5312, -78.725) centre (256.5312, -79.225) ccw
  arc A310 (243.0313, -92.225) -> (243.5313, -92.725) centre (243.5313, -92.225) ccw
  arc A311 (256.5312, -92.725) -> (257.0312, -92.225) centre (256.5312, -92.225) ccw
  line L312 (269.725, -78.725) -> (282.725, -78.725)
  line L313 (269.725, -92.725) -> (282.725, -92.725)
  line L314 (269.225, -79.225) -> (269.225, -92.225)
  line L315 (283.225, -79.225) -> (283.225, -92.225)
  arc A312 (269.725, -78.725) -> (269.225, -79.225) centre (269.725, -79.225) ccw
  arc A313 (283.225, -79.225) -> (282.725, -78.725) centre (282.725, -79.225) ccw
  arc A314 (269.225, -92.225) -> (269.725, -92.725) centre (269.725, -92.225) ccw
  arc A315 (282.725, -92.725) -> (283.225, -92.225) centre (282.725, -92.225) ccw
  line L316 (288.775, -78.725) -> (301.775, -78.725)
  line L317 (288.775, -92.725) -> (301.775, -92.725)
  line L318 (288.275, -79.225) -> (288.275, -92.225)
  line L319 (302.275, -79.225) -> (302.275, -92.225)
  arc A316 (288.775, -78.725) -> (288.275, -79.225) centre (288.775, -79.225) ccw
  arc A317 (302.275, -79.225) -> (301.775, -78.725) centre (301.775, -79.225) ccw